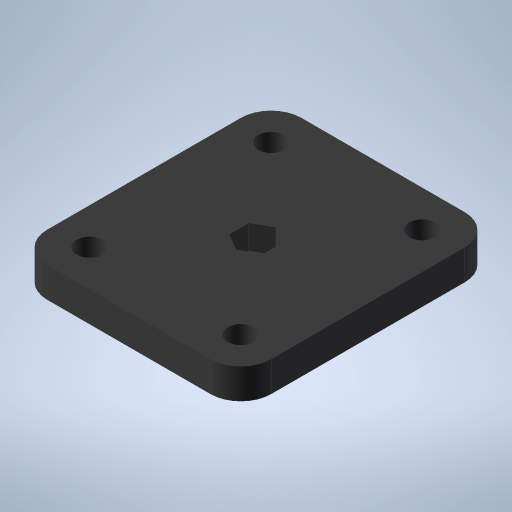
# Autodesk Inventor part: Yagi_fixed_plate
Saved by Autodesk Inventor 2023 (Build 270158000, 158)
## iProperties
Created: 2023-09-05
Part Number: Yagi_fixed_plate
Material: 一般
Document SubType Name: Modeling
Designer: 310611102
Density: 1 g/cm^3
Appearance: 預設
Author: 310611102
Autodesk Inventor part; units mm, degrees
ref_plane "YZ Plane" through (0, 0, 0) normal (1, 0, 0) x (0, 1, 0)
ref_plane "XZ Plane" through (0, 0, 0) normal (0, 1, 0) x (-1, 0, 0)
ref_plane "XY Plane" through (0, 0, 0) normal (0, 0, 1) x (1, 0, 0)
sketch "Sketch1" plane through (0, 0, 0) normal (0, 1, 0) x (-1, 0, 0)
  line L0 (37, 42) -> (-37, 42)
  line L1 (-37, 42) -> (-37, -42)
  line L2 (-37, -42) -> (37, -42)
  line L3 (37, -42) -> (37, 42)
  line L4 (37, 42) -> (-37, -42) construction
  line L5 (-37, 42) -> (37, -42) construction
  circle A0 centre (25, 30) radius 4.35
  circle A1 centre (25, -30) radius 4.35
  circle A2 centre (-25, 30) radius 4.35
  circle A3 centre (-25, -30) radius 4.35
  point P0 (0, 0)
  dimension "d0" = 74
  dimension "d1" = 84
  dimension "d4" = 60
  dimension "d7" = 50
  dimension "d10" = 8.7
  dimension "d11" = 12
  dimension "d12" = 12
  constraints: 12 end point, 4 centre point, 2 horizontal, 2 midpoint, 2 parallel, 1 perpendicular, 1 vertical, 6 other
  measures "d0" distance of L1.end L2.end
  measures "d1" distance of L2.end L0.start
  measures "d4" distance of A0.centre A1.centre
  measures "d7" distance of A0.centre A2.centre
  measures "d10" diameter of A0
  measures "d11" distance from line of L0 A0.centre
  measures "d12" distance from line of L3 A0.centre
extrude "Extrusion1" add sketch "Sketch1" along normal blind 10
fillet "Fillet1" radius 10 4 edges at (-37, 5, 42) (37, 5, 42) (37, 5, -42) (-37, 5, -42)
sketch "Sketch2" plane through (0, 10, 0) normal (0, 1, 0) x (1, 0, 0)
  line L0 (0, 6.5241) -> (5.65, 3.262)
  line L1 (5.65, 3.262) -> (5.65, -3.262)
  line L2 (5.65, -3.262) -> (0, -6.5241)
  line L3 (0, -6.5241) -> (-5.65, -3.262)
  line L4 (-5.65, -3.262) -> (-5.65, 3.262)
  line L5 (-5.65, 3.262) -> (0, 6.5241)
  point P0 (0, 0)
  point P1 (0, 0)
  dimension "d16" = 11.3
  constraints: 12 end point, 1 coincident, 1 vertical alignment, 13 other
  measures "d16" distance between parallel lines of L1 L4
extrude "Extrusion2" cut sketch "Sketch2" against normal blind 8
sketch "Sketch3" plane through (0, 2, 0) normal (0, 1, 0) x (1, 0, 0)
  circle A0 centre (0, 0) radius 3.5
  dimension "d19" = 7
  constraints: 1 centre point, 1 coincident
  measures "d19" diameter of A0
extrude "Extrusion3" cut sketch "Sketch3" against normal through all
body "Solid1"
